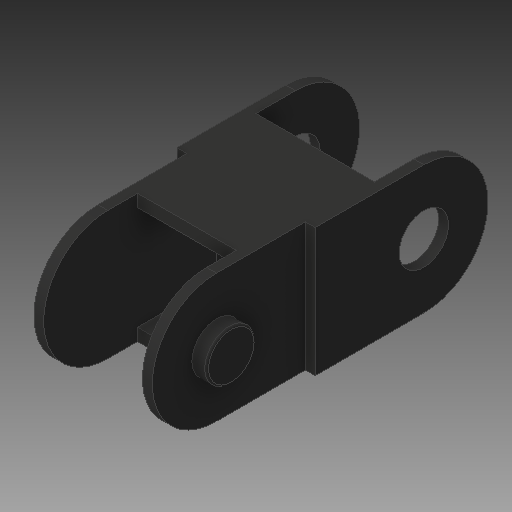
# Autodesk Inventor part: Esteira-fesma-S10
Saved by Autodesk Inventor 2017 (Build 210142000, 142)
## iProperties
Created: 2016-07-07
Part Number: Esteira-fesma-S10
Material: Nylon 6/6
Document SubType Name: Modeling
Designer: hmigu
Density: 1.13 g/cm^3
Appearance: Rubber - Black
Author: hmigu
Autodesk Inventor part; units mm, degrees
ref_plane "YZ Plane" through (0, 0, 0) normal (1, 0, 0) x (0, 1, 0)
ref_plane "XZ Plane" through (0, 0, 0) normal (0, 1, 0) x (-1, 0, 0)
ref_plane "XY Plane" through (0, 0, 0) normal (0, 0, 1) x (1, 0, 0)
sketch "Sketch1" plane through (0, 0, 0) normal (0, 1, 0) x (-1, 0, 0)
  line L0 (-5, 16.5) -> (-5, -1)
  line L1 (-5, -1) -> (-6, -1)
  line L2 (-6, -1) -> (-6, -16.5)
  line L3 (-6, -16.5) -> (-7, -16.5)
  line L4 (-7, -16.5) -> (-7, 1)
  line L5 (-7, 1) -> (-6, 1)
  line L6 (-6, 1) -> (-6, 16.5)
  line L7 (-6, 16.5) -> (-5, 16.5)
  line L8 (0, 14.862) -> (0, -14.862)
  line L9 (-6, 1) -> (-6, -1) construction
  point P0 (0, 0)
  point P1 (0, 0)
  point P2 (-6, 0)
  dimension "d0" = 12
  dimension "d1" = 10
  dimension "d2" = 33
  dimension "d3" = 2
  dimension "d20" = 1
  constraints: 20 end point, 6 perpendicular, 3 vertical, 2 midpoint, 2 point on line, 1 coincident, 1 horizontal alignment, 1 parallel
  measures "d0" diameter of L6 L8
  measures "d1" diameter of L0 L8
  measures "d2" distance from line of L3.end L7
  measures "d3" distance of L5.end L1.end
  measures "d20" distance of L2.end L3.end
extrude "Extrusion1" add sketch "Sketch1" along normal mid plane 13
sketch "Sketch2" plane through (7, -6.5, -16.5) normal (1, 0, 0) x (0, 0, -1)
  arc A0 (-26.5, 13) -> (-26.5, 0) centre (-26.5, 6.5) ccw
  line L0 (-17.5, 13) -> (-17.5, 0) projected
  line L1 (-33, 13) -> (-17.5, 13) projected
  line L2 (-33, 13) -> (-33, 0) projected
  line L3 (-17.5, 0) -> (-33, 0) projected
  line L4 (0, 13) -> (0, 0) projected
  line L5 (-17.5, 13) -> (0, 13) projected
  line L6 (-17.5, 13) -> (-17.5, 0) projected
  line L7 (0, 0) -> (-17.5, 0) projected
  arc A1 (-6.5, 0) -> (-6.5, 13) centre (-6.5, 6.5) ccw
  circle A2 centre (-6.5, 6.5) radius 2.5
  circle A3 centre (-26.5, 6.5) radius 2.5
  line L8 (-15.5, 13) -> (-33, 13) projected
  line L9 (-26.5, 13) -> (-33, 13)
  line L10 (-33, 13) -> (-33, 0)
  line L11 (0, 0) -> (-17.5, 0) projected
  line L12 (-6.5, 0) -> (0, 0)
  line L13 (0, 0) -> (0, 13)
  line L14 (-17.5, 13) -> (0, 13) projected
  line L15 (-6.5, 13) -> (0, 13)
  point P0 (-16.5, 6.5)
  dimension "d6" = 5
  dimension "d7" = 5
  constraints: 10 end point, 8 tangent, 4 centre point, 4 point on circle, 4 point on line, 3 collinear, 2 coincident, 1 horizontal, 1 perpendicular
  measures "d6" diameter of A2
  measures "d7" diameter of A3
extrude "Extrusion2" cut sketch "Sketch2" against normal through all contours A0 L2 L1 | A0 L3 L2 | A1 L4 L7 | L5 L4 A1 | A2
extrude "Extrusion3" add sketch "Sketch2" along normal blind 0.5 and the other way blind 1.5 contours A3
ref_plane "Work Plane1" through (0, -6.5, -1) normal (-1, 0, 0) x (0, 0, 1)
mirror "Mirror1" about plane through (0, -6.5, -1) normal (-1, 0, 0)
sketch "Sketch3" plane through (6, -6.5, -1) normal (-1, 0, 0) x (0, 0, 1)
  line L0 (2, 13) -> (-9, 13) projected
  line L1 (-5, 13) -> (8, 13)
  line L2 (8, 13) -> (8, 11.75)
  line L3 (8, 11.75) -> (-5, 11.75)
  line L4 (-5, 11.75) -> (-5, 13)
  circle A0 centre (-9, 6.5) radius 2.5 projected
  circle A1 centre (11, 6.5) radius 2.5 projected
  line L5 (-9, 0) -> (2, 0) projected
  line L6 (-5, 0) -> (8, 0)
  line L7 (8, 0) -> (8, 1.25)
  line L8 (8, 1.25) -> (-5, 1.25)
  line L9 (-5, 1.25) -> (-5, 0)
  point P0 (1, 6.5)
  dimension "d15" = 4
  dimension "d16" = 10.5
  dimension "d17" = 3
  constraints: 16 end point, 4 parallel, 3 collinear, 2 horizontal, 2 perpendicular, 2 point on line
  measures "d15" distance from line of A0.centre L4
  measures "d16" distance between parallel lines of L8 L3
  measures "d17" distance from line of L2 A1.centre
extrude "Extrusion4" add sketch "Sketch3" along normal up to surface (12 mm away) contours L1 L2 L3 L4 L0 | L9 L8 L7 L6 L5
fillet "Fillet1" radius 0.2 2 edges at (7.5, 0, 12.5) (-7.5, 0, 12.5)
body "Solid1"
